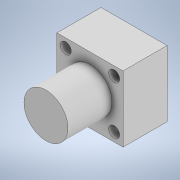
# Autodesk Inventor part: bottom piece pvc
Saved by Autodesk Inventor 2020 (Build 240168000, 168)
## iProperties
Created: 2020-01-25
Part Number: bottom piece pvc
Material: Generic
Document SubType Name: Modeling
Designer: 1jyng
Density: 1 g/cm^3
Appearance: Default
Author: 1jyng
Autodesk Inventor part; units mm, degrees
ref_plane "YZ Plane" through (0, 0, 0) normal (1, 0, 0) x (0, 1, 0)
ref_plane "XZ Plane" through (0, 0, 0) normal (0, 1, 0) x (-1, 0, 0)
ref_plane "XY Plane" through (0, 0, 0) normal (0, 0, 1) x (1, 0, 0)
sketch "Sketch1" plane through (0, 0, 0) normal (0, 0, 1) x (1, 0, 0)
  line L0 (-6.0176, 0) -> (13.0324, 0)
  line L1 (13.0324, 0) -> (13.0324, 19.05)
  line L2 (13.0324, 19.05) -> (-6.0176, 19.05)
  line L3 (-6.0176, 19.05) -> (-6.0176, 0)
  point P0 (0, 0)
  dimension "d0" = 19.05
  dimension "d1" = 19.05
  constraints: 8 end point, 2 parallel, 1 horizontal, 1 perpendicular
  measures "d0" distance of L0.end L1.end
  measures "d1" distance of L0.start L0.end
extrude "Extrusion1" add sketch "Sketch1" along normal blind 12.7
sketch "Sketch2" plane through (0, 0, 12.7) normal (0, 0, 1) x (1, 0, 0)
  circle A0 centre (3.5074, 9.525) radius 6.35
  line L0 (13.0324, 19.05) -> (-6.0176, 19.05) projected
  line L1 (13.0324, 0) -> (13.0324, 19.05) projected
  circle A1 centre (10.4924, 16.51) radius 1.5875
  circle A2 centre (10.4924, 2.54) radius 1.5875
  line L2 (-6.0176, 0) -> (13.0324, 0) projected
  circle A3 centre (-3.4776, 16.51) radius 1.5875
  line L3 (-6.0176, 19.05) -> (-6.0176, 0) projected
  circle A4 centre (-3.4776, 2.54) radius 1.5875
  point P0 (0, 0)
  dimension "d4" = 9.525
  dimension "d5" = 9.525
  dimension "d6" = 12.7
  dimension "d9" = 3.175
  dimension "d10" = 2.54
  dimension "d11" = 2.54
  dimension "d12" = 3.175
  dimension "d13" = 2.54
  dimension "d14" = 2.54
  dimension "d15" = 3.175
  dimension "d16" = 2.54
  dimension "d17" = 2.54
  dimension "d18" = 3.175
  dimension "d19" = 2.54
  dimension "d20" = 2.54
  constraints: 5 centre point
  measures "d4" distance from line of L0 A0.centre
  measures "d5" distance from line of L1 A0.centre
  measures "d6" diameter of A0
  measures "d9" diameter of A1
  measures "d10" distance from line of L0 A1.centre
  measures "d11" distance from line of L1 A1.centre
  measures "d12" diameter of A2
  measures "d13" distance from line of L1 A2.centre
  measures "d14" distance from line of L2 A2.centre
  measures "d15" diameter of A3
  measures "d16" distance from line of L0 A3.centre
  measures "d17" distance from line of L3 A3.centre
  measures "d18" diameter of A4
  measures "d19" distance from line of L2 A4.centre
  measures "d20" distance from line of L3 A4.centre
extrude "Extrusion2" add sketch "Sketch2" along normal blind 12.7 contours A0
sketch "Sketch3" plane through (0, 0, 12.7) normal (0, 0, 1) x (1, 0, 0)
  circle A0 centre (10.4924, 16.51) radius 1.5875
  circle A1 centre (-3.4776, 16.51) radius 1.5875
  circle A2 centre (-3.4776, 2.54) radius 1.5875
  circle A3 centre (10.4924, 2.54) radius 1.5875
  line L0 (-6.0176, 0) -> (13.0324, 0) projected
  line L1 (-6.0176, 19.05) -> (-6.0176, 0) projected
  line L2 (13.0324, 19.05) -> (-6.0176, 19.05) projected
  line L3 (13.0324, 0) -> (13.0324, 19.05) projected
  point P0 (0, 0)
  dimension "d21" = 3.175
  dimension "d22" = 3.175
  dimension "d23" = 3.175
  dimension "d24" = 3.175
  dimension "d25" = 2.54
  dimension "d26" = 2.54
  dimension "d27" = 2.54
  dimension "d28" = 2.54
  dimension "d29" = 2.54
  dimension "d30" = 2.54
  dimension "d31" = 2.54
  dimension "d32" = 2.54
  constraints: 4 centre point
  measures "d21" diameter of A0
  measures "d22" diameter of A3
  measures "d23" diameter of A1
  measures "d24" diameter of A2
  measures "d25" distance from line of A2.centre L0
  measures "d26" distance from line of L1 A2.centre
  measures "d27" distance from line of L2 A1.centre
  measures "d28" distance from line of L1 A1.centre
  measures "d29" distance from line of L2 A0.centre
  measures "d30" distance from line of L3 A0.centre
  measures "d31" distance from line of L0 A3.centre
  measures "d32" distance from line of L3 A3.centre
extrude "Extrusion3" cut sketch "Sketch3" against normal blind 12.7 contours A0 | A1 | A2 | A3
body "Solid1"
